Autodesk Fusion 360 part; units mm, degrees
note: some values were not read from the file. Chosen so that the rebuilt part matches the saved one: a direction. Set by a fixed rule: which sketch regions a step uses; which face or edge a step refers to.
(part 5 of 6)
  line L1273 (135.5672, -17.489) -> (135.5672, -15.9015)
  spline S993 degree 3 poles (135.5672, -15.9015) (135.5672, -15.8869) (135.5553, -15.875) (135.5408, -15.875) knots 0 0 0 0 1 1 1 1
  line L1274 (135.5408, -15.875) -> (135.1703, -15.875)
  spline S994 degree 3 poles (135.1703, -15.875) (135.1439, -15.875) (135.1703, -15.9015) (135.1703, -15.875) knots 0 0 0 0 1 1 1 1
  line L1275 (135.1703, -15.875) -> (135.1703, -14.3404)
  spline S995 degree 3 poles (135.1703, -14.3404) (135.1703, -14.314) (135.1439, -14.3404) (135.1703, -14.3404) knots 0 0 0 0 1 1 1 1
  line L1276 (135.1703, -14.3404) -> (135.5408, -14.3404)
  spline S996 degree 3 poles (135.5408, -14.3404) (135.5553, -14.3404) (135.5672, -14.3285) (135.5672, -14.314) knots 0 0 0 0 1 1 1 1
  line L1277 (135.5672, -14.314) -> (135.5672, -12.7265)
  spline S997 degree 3 poles (135.5672, -12.7265) (135.5672, -12.7119) (135.5553, -12.7) (135.5408, -12.7) knots 0 0 0 0 1 1 1 1
  line L1278 (135.5408, -12.7) -> (135.1703, -12.7)
  spline S998 degree 3 poles (135.1703, -12.7) (135.1439, -12.7) (135.1703, -12.7265) (135.1703, -12.7) knots 0 0 0 0 1 1 1 1
  line L1279 (135.1703, -12.7) -> (135.1703, -11.1654)
  spline S999 degree 3 poles (135.1703, -11.1654) (135.1703, -11.139) (135.1439, -11.1654) (135.1703, -11.1654) knots 0 0 0 0 1 1 1 1
  line L1280 (135.1703, -11.1654) -> (135.5408, -11.1654)
  spline S1000 degree 3 poles (135.5408, -11.1654) (135.5553, -11.1654) (135.5672, -11.1535) (135.5672, -11.139) knots 0 0 0 0 1 1 1 1
  line L1281 (135.5672, -11.139) -> (135.5672, -9.5515)
  spline S1001 degree 3 poles (135.5672, -9.5515) (135.5672, -9.5369) (135.5553, -9.525) (135.5408, -9.525) knots 0 0 0 0 1 1 1 1
  line L1282 (135.5408, -9.525) -> (135.1703, -9.525)
  spline S1002 degree 3 poles (135.1703, -9.525) (135.1439, -9.525) (135.1703, -9.5515) (135.1703, -9.525) knots 0 0 0 0 1 1 1 1
  line L1283 (135.1703, -9.525) -> (135.1703, -7.9904)
  spline S1003 degree 3 poles (135.1703, -7.9904) (135.1703, -7.964) (135.1439, -7.9904) (135.1703, -7.9904) knots 0 0 0 0 1 1 1 1
  line L1284 (135.1703, -7.9904) -> (135.5408, -7.9904)
  spline S1004 degree 3 poles (135.5408, -7.9904) (135.5553, -7.9904) (135.5672, -7.9785) (135.5672, -7.964) knots 0 0 0 0 1 1 1 1
  line L1285 (135.5672, -7.964) -> (135.5672, -6.3765)
  spline S1005 degree 3 poles (135.5672, -6.3765) (135.5672, -6.3619) (135.5553, -6.35) (135.5408, -6.35) knots 0 0 0 0 1 1 1 1
  line L1286 (135.5408, -6.35) -> (135.1703, -6.35)
  spline S1006 degree 3 poles (135.1703, -6.35) (135.1439, -6.35) (135.1703, -6.3765) (135.1703, -6.35) knots 0 0 0 0 1 1 1 1
  line L1287 (135.1703, -6.35) -> (135.1703, -3.466)
  spline S1007 degree 3 poles (135.1703, -3.466) (135.1703, -3.4515) (135.1584, -3.4396) (135.1439, -3.4396) knots 0 0 0 0 1 1 1 1
  line L1288 (135.1439, -3.4396) -> (135.328, -3.4396)
  line L1289 (135.328, -3.4396) -> (133.9226, -3.4396)
  spline S1008 degree 3 poles (133.9226, -3.4396) (133.8961, -3.4396) (133.9226, -3.466) (133.9226, -3.4396) knots 0 0 0 0 1 1 1 1
  line L1290 (133.9226, -3.4396) -> (133.9226, -2.6723)
  spline S1009 degree 3 poles (133.9226, -2.6723) (133.9226, -2.6577) (133.9109, -2.6458) (133.8961, -2.6458) knots 0 0 0 0 1 1 1 1
  line L1291 (133.8961, -2.6458) -> (132.3086, -2.6458)
  spline S1010 degree 3 poles (132.3086, -2.6458) (132.294, -2.6458) (132.2821, -2.6577) (132.2821, -2.6723) knots 0 0 0 0 1 1 1 1
  line L1292 (132.2821, -2.6723) -> (132.2821, -3.4396)
  spline S1011 degree 3 poles (132.2821, -3.4396) (132.2821, -3.466) (132.3086, -3.4396) (132.2821, -3.4396) knots 0 0 0 0 1 1 1 1
  line L1293 (132.2821, -3.4396) -> (130.8769, -3.4396)
  line L1294 (130.8769, -3.4396) -> (130.6642, -3.4396)
  spline S1012 degree 3 poles (130.6642, -3.4396) (130.6497, -3.4396) (130.6378, -3.4515) (130.6378, -3.466) knots 0 0 0 0 1 1 1 1
  line L1295 (130.6378, -3.466) -> (130.6378, -6.3765)
  spline S1013 degree 3 poles (130.6378, -6.3765) (130.6378, -6.391) (130.6497, -6.4029) (130.6642, -6.4029) knots 0 0 0 0 1 1 1 1
  line L1296 (130.6642, -6.4029) -> (131.0346, -6.4029)
  spline S1014 degree 3 poles (131.0346, -6.4029) (131.0611, -6.4029) (131.0346, -6.3765) (131.0346, -6.4029) knots 0 0 0 0 1 1 1 1
  line L1297 (131.0346, -6.4029) -> (131.0346, -7.9375)
  spline S1015 degree 3 poles (131.0346, -7.9375) (131.0346, -7.964) (131.0611, -7.9375) (131.0346, -7.9375) knots 0 0 0 0 1 1 1 1
  line L1298 (131.0346, -7.9375) -> (130.6642, -7.9375)
  spline S1016 degree 3 poles (130.6642, -7.9375) (130.6497, -7.9375) (130.6378, -7.9494) (130.6378, -7.964) knots 0 0 0 0 1 1 1 1
  line L1299 (130.6378, -7.964) -> (130.6378, -9.5515)
  spline S1017 degree 3 poles (130.6378, -9.5515) (130.6378, -9.566) (130.6497, -9.5779) (130.6642, -9.5779) knots 0 0 0 0 1 1 1 1
  line L1300 (130.6642, -9.5779) -> (131.0346, -9.5779)
  spline S1018 degree 3 poles (131.0346, -9.5779) (131.0611, -9.5779) (131.0346, -9.5515) (131.0346, -9.5779) knots 0 0 0 0 1 1 1 1
  line L1301 (131.0346, -9.5779) -> (131.0346, -11.1125)
  spline S1019 degree 3 poles (131.0346, -11.1125) (131.0346, -11.139) (131.0611, -11.1125) (131.0346, -11.1125) knots 0 0 0 0 1 1 1 1
  line L1302 (131.0346, -11.1125) -> (130.6642, -11.1125)
  spline S1020 degree 3 poles (130.6642, -11.1125) (130.6497, -11.1125) (130.6378, -11.1244) (130.6378, -11.139) knots 0 0 0 0 1 1 1 1
  line L1303 (130.6378, -11.139) -> (130.6378, -12.7265)
  spline S1021 degree 3 poles (130.6378, -12.7265) (130.6378, -12.741) (130.6497, -12.7529) (130.6642, -12.7529) knots 0 0 0 0 1 1 1 1
  line L1304 (130.6642, -12.7529) -> (131.0346, -12.7529)
  spline S1022 degree 3 poles (131.0346, -12.7529) (131.0611, -12.7529) (131.0346, -12.7265) (131.0346, -12.7529) knots 0 0 0 0 1 1 1 1
  line L1305 (131.0346, -12.7529) -> (131.0346, -14.2875)
  spline S1023 degree 3 poles (131.0346, -14.2875) (131.0346, -14.314) (131.0611, -14.2875) (131.0346, -14.2875) knots 0 0 0 0 1 1 1 1
  line L1306 (131.0346, -14.2875) -> (130.6642, -14.2875)
  spline S1024 degree 3 poles (130.6642, -14.2875) (130.6497, -14.2875) (130.6378, -14.2994) (130.6378, -14.314) knots 0 0 0 0 1 1 1 1
  line L1307 (130.6378, -14.314) -> (130.6378, -15.9015)
  spline S1025 degree 3 poles (130.6378, -15.9015) (130.6378, -15.916) (130.6497, -15.9279) (130.6642, -15.9279) knots 0 0 0 0 1 1 1 1
  line L1308 (130.6642, -15.9279) -> (131.0346, -15.9279)
  spline S1026 degree 3 poles (131.0346, -15.9279) (131.0611, -15.9279) (131.0346, -15.9015) (131.0346, -15.9279) knots 0 0 0 0 1 1 1 1
  line L1309 (131.0346, -15.9279) -> (131.0346, -17.4625)
  spline S1027 degree 3 poles (131.0346, -17.4625) (131.0346, -17.489) (131.0611, -17.4625) (131.0346, -17.4625) knots 0 0 0 0 1 1 1 1
  line L1310 (131.0346, -17.4625) -> (130.6642, -17.4625)
  spline S1028 degree 3 poles (130.6642, -17.4625) (130.6497, -17.4625) (130.6378, -17.4744) (130.6378, -17.489) knots 0 0 0 0 1 1 1 1
  line L1311 (130.6378, -17.489) -> (130.6378, -19.0765)
  spline S1029 degree 3 poles (130.6378, -19.0765) (130.6378, -19.091) (130.6497, -19.1029) (130.6642, -19.1029) knots 0 0 0 0 1 1 1 1
  line L1312 (130.6642, -19.1029) -> (131.0346, -19.1029)
  spline S1030 degree 3 poles (131.0346, -19.1029) (131.0611, -19.1029) (131.0346, -19.0765) (131.0346, -19.1029) knots 0 0 0 0 1 1 1 1
  line L1313 (131.0346, -19.1029) -> (131.0346, -20.6375)
  spline S1031 degree 3 poles (131.0346, -20.6375) (131.0346, -20.664) (131.0611, -20.6375) (131.0346, -20.6375) knots 0 0 0 0 1 1 1 1
  line L1314 (131.0346, -20.6375) -> (130.6642, -20.6375)
  spline S1032 degree 3 poles (130.6642, -20.6375) (130.6497, -20.6375) (130.6378, -20.6494) (130.6378, -20.664) knots 0 0 0 0 1 1 1 1
  line L1315 (130.6378, -20.664) -> (130.6378, -22.2515)
  spline S1033 degree 3 poles (130.6378, -22.2515) (130.6378, -22.266) (130.6497, -22.2779) (130.6642, -22.2779) knots 0 0 0 0 1 1 1 1
  line L1316 (130.6642, -22.2779) -> (131.0346, -22.2779)
  spline S1034 degree 3 poles (131.0346, -22.2779) (131.0611, -22.2779) (131.0346, -22.2515) (131.0346, -22.2779) knots 0 0 0 0 1 1 1 1
  line L1317 (131.0346, -22.2779) -> (131.0346, -23.8125)
  spline S1035 degree 3 poles (131.0346, -23.8125) (131.0346, -23.839) (131.0611, -23.8125) (131.0346, -23.8125) knots 0 0 0 0 1 1 1 1
  line L1318 (131.0346, -23.8125) -> (130.6642, -23.8125)
  spline S1036 degree 3 poles (130.6642, -23.8125) (130.6497, -23.8125) (130.6378, -23.8244) (130.6378, -23.839) knots 0 0 0 0 1 1 1 1
  line L1319 (130.6378, -23.839) -> (130.6378, -25.4265)
  spline S1037 degree 3 poles (130.6378, -25.4265) (130.6378, -25.441) (130.6497, -25.4529) (130.6642, -25.4529) knots 0 0 0 0 1 1 1 1
  line L1320 (130.6642, -25.4529) -> (131.0346, -25.4529)
  spline S1038 degree 3 poles (131.0346, -25.4529) (131.0611, -25.4529) (131.0346, -25.4265) (131.0346, -25.4529) knots 0 0 0 0 1 1 1 1
  line L1321 (131.0346, -25.4529) -> (131.0346, -26.9875)
  spline S1039 degree 3 poles (131.0346, -26.9875) (131.0346, -27.014) (131.0611, -26.9875) (131.0346, -26.9875) knots 0 0 0 0 1 1 1 1
  line L1322 (131.0346, -26.9875) -> (130.6642, -26.9875)
  spline S1040 degree 3 poles (130.6642, -26.9875) (130.6497, -26.9875) (130.6378, -26.9994) (130.6378, -27.014) knots 0 0 0 0 1 1 1 1
  line L1323 (130.6378, -27.014) -> (130.6378, -29.9244)
  spline S1041 degree 3 poles (130.6378, -29.9244) (130.6378, -29.9389) (130.6497, -29.9508) (130.6642, -29.9508) knots 0 0 0 0 1 1 1 1
  line L1324 (130.6642, -29.9508) -> (130.8769, -29.9508)
  line L1325 (136.2033, -29.9508) -> (137.6085, -29.9508)
  spline S1042 degree 3 poles (137.6085, -29.9508) (137.6349, -29.9508) (137.6085, -29.9244) (137.6085, -29.9508) knots 0 0 0 0 1 1 1 1
  line L1326 (137.6085, -29.9508) -> (137.6085, -30.7181)
  spline S1043 degree 3 poles (137.6085, -30.7181) (137.6085, -30.7327) (137.6204, -30.7446) (137.6349, -30.7446) knots 0 0 0 0 1 1 1 1
  line L1327 (137.6349, -30.7446) -> (139.2224, -30.7446)
  spline S1044 degree 3 poles (139.2224, -30.7446) (139.237, -30.7446) (139.2489, -30.7327) (139.2489, -30.7181) knots 0 0 0 0 1 1 1 1
  line L1328 (139.2489, -30.7181) -> (139.2489, -29.9508)
  spline S1045 degree 3 poles (139.2489, -29.9508) (139.2489, -29.9244) (139.2224, -29.9508) (139.2489, -29.9508) knots 0 0 0 0 1 1 1 1
  line L1329 (139.2489, -29.9508) -> (140.6544, -29.9508)
  line L1330 (140.6544, -29.9508) -> (140.5533, -29.9508)
  spline S1046 degree 3 poles (140.5533, -29.9508) (140.5681, -29.9508) (140.5797, -29.9389) (140.5797, -29.9244) knots 0 0 0 0 1 1 1 1
  line L1331 (140.5797, -29.9244) -> (140.5797, -27.0404)
  spline S1047 degree 3 poles (140.5797, -27.0404) (140.5797, -27.014) (140.5533, -27.0404) (140.5797, -27.0404) knots 0 0 0 0 1 1 1 1
  line L1332 (140.5797, -27.0404) -> (140.7589, -27.0404)
  spline S1048 degree 3 poles (140.7589, -27.0404) (140.7734, -27.0404) (140.7853, -27.0285) (140.7853, -27.014) knots 0 0 0 0 1 1 1 1
  line L1333 (140.7853, -27.014) -> (140.7853, -25.4265)
  spline S1049 degree 3 poles (140.7853, -25.4265) (140.7853, -25.4119) (140.7734, -25.4) (140.7589, -25.4) knots 0 0 0 0 1 1 1 1
  line L1334 (140.7589, -25.4) -> (140.5797, -25.4)
  spline S1050 degree 3 poles (140.5797, -25.4) (140.5533, -25.4) (140.5797, -25.4265) (140.5797, -25.4) knots 0 0 0 0 1 1 1 1
  line L1335 (140.5797, -25.4) -> (140.5797, -23.8654)
  spline S1051 degree 3 poles (140.5797, -23.8654) (140.5797, -23.839) (140.5533, -23.8654) (140.5797, -23.8654) knots 0 0 0 0 1 1 1 1
  line L1336 (140.5797, -23.8654) -> (140.7589, -23.8654)
  spline S1052 degree 3 poles (140.7589, -23.8654) (140.7734, -23.8654) (140.7853, -23.8535) (140.7853, -23.839) knots 0 0 0 0 1 1 1 1
  line L1337 (140.7853, -23.839) -> (140.7853, -22.2515)
  spline S1053 degree 3 poles (140.7853, -22.2515) (140.7853, -22.2369) (140.7734, -22.225) (140.7589, -22.225) knots 0 0 0 0 1 1 1 1
  line L1338 (140.7589, -22.225) -> (140.5797, -22.225)
  spline S1054 degree 3 poles (140.5797, -22.225) (140.5533, -22.225) (140.5797, -22.2515) (140.5797, -22.225) knots 0 0 0 0 1 1 1 1
  line L1339 (140.5797, -22.225) -> (140.5797, -20.6904)
  spline S1055 degree 3 poles (140.5797, -20.6904) (140.5797, -20.664) (140.5533, -20.6904) (140.5797, -20.6904) knots 0 0 0 0 1 1 1 1
  line L1340 (140.5797, -20.6904) -> (140.7589, -20.6904)
  spline S1056 degree 3 poles (140.7589, -20.6904) (140.7734, -20.6904) (140.7853, -20.6785) (140.7853, -20.664) knots 0 0 0 0 1 1 1 1
  line L1341 (140.7853, -20.664) -> (140.7853, -19.0765)
  spline S1057 degree 3 poles (140.7853, -19.0765) (140.7853, -19.0619) (140.7734, -19.05) (140.7589, -19.05) knots 0 0 0 0 1 1 1 1
  line L1342 (140.7589, -19.05) -> (140.5797, -19.05)
  spline S1058 degree 3 poles (140.5797, -19.05) (140.5533, -19.05) (140.5797, -19.0765) (140.5797, -19.05) knots 0 0 0 0 1 1 1 1
  line L1343 (140.5797, -19.05) -> (140.5797, -17.5154)
  spline S1059 degree 3 poles (140.5797, -17.5154) (140.5797, -17.489) (140.5533, -17.5154) (140.5797, -17.5154) knots 0 0 0 0 1 1 1 1
  line L1344 (140.5797, -17.5154) -> (140.7589, -17.5154)
  spline S1060 degree 3 poles (140.7589, -17.5154) (140.7734, -17.5154) (140.7853, -17.5035) (140.7853, -17.489) knots 0 0 0 0 1 1 1 1
  line L1345 (140.7853, -17.489) -> (140.7853, -15.9015)
  spline S1061 degree 3 poles (140.7853, -15.9015) (140.7853, -15.8869) (140.7734, -15.875) (140.7589, -15.875) knots 0 0 0 0 1 1 1 1
  line L1346 (140.7589, -15.875) -> (140.5797, -15.875)
  spline S1062 degree 3 poles (140.5797, -15.875) (140.5533, -15.875) (140.5797, -15.9015) (140.5797, -15.875) knots 0 0 0 0 1 1 1 1
  line L1347 (140.5797, -15.875) -> (140.5797, -14.3404)
  spline S1063 degree 3 poles (140.5797, -14.3404) (140.5797, -14.314) (140.5533, -14.3404) (140.5797, -14.3404) knots 0 0 0 0 1 1 1 1
  line L1348 (140.5797, -14.3404) -> (140.7589, -14.3404)
  spline S1064 degree 3 poles (140.7589, -14.3404) (140.7734, -14.3404) (140.7853, -14.3285) (140.7853, -14.314) knots 0 0 0 0 1 1 1 1
  line L1349 (140.7853, -14.314) -> (140.7853, -12.7265)
  spline S1065 degree 3 poles (140.7853, -12.7265) (140.7853, -12.7119) (140.7734, -12.7) (140.7589, -12.7) knots 0 0 0 0 1 1 1 1
  line L1350 (140.7589, -12.7) -> (140.5797, -12.7)
  spline S1066 degree 3 poles (140.5797, -12.7) (140.5533, -12.7) (140.5797, -12.7265) (140.5797, -12.7) knots 0 0 0 0 1 1 1 1
  line L1351 (140.5797, -12.7) -> (140.5797, -11.1654)
  spline S1067 degree 3 poles (140.5797, -11.1654) (140.5797, -11.139) (140.5533, -11.1654) (140.5797, -11.1654) knots 0 0 0 0 1 1 1 1
  line L1352 (140.5797, -11.1654) -> (140.7589, -11.1654)
  spline S1068 degree 3 poles (140.7589, -11.1654) (140.7734, -11.1654) (140.7853, -11.1535) (140.7853, -11.139) knots 0 0 0 0 1 1 1 1
  line L1353 (140.7853, -11.139) -> (140.7853, -9.5515)
  spline S1069 degree 3 poles (140.7853, -9.5515) (140.7853, -9.5369) (140.7734, -9.525) (140.7589, -9.525) knots 0 0 0 0 1 1 1 1
  line L1354 (140.7589, -9.525) -> (140.5797, -9.525)
  spline S1070 degree 3 poles (140.5797, -9.525) (140.5533, -9.525) (140.5797, -9.5515) (140.5797, -9.525) knots 0 0 0 0 1 1 1 1
  line L1355 (140.5797, -9.525) -> (140.5797, -7.9904)
  spline S1071 degree 3 poles (140.5797, -7.9904) (140.5797, -7.964) (140.5533, -7.9904) (140.5797, -7.9904) knots 0 0 0 0 1 1 1 1
  line L1356 (140.5797, -7.9904) -> (140.7589, -7.9904)
  spline S1072 degree 3 poles (140.7589, -7.9904) (140.7734, -7.9904) (140.7853, -7.9785) (140.7853, -7.964) knots 0 0 0 0 1 1 1 1
  line L1357 (140.7853, -7.964) -> (140.7853, -6.3765)
  spline S1073 degree 3 poles (140.7853, -6.3765) (140.7853, -6.3619) (140.7734, -6.35) (140.7589, -6.35) knots 0 0 0 0 1 1 1 1
  line L1358 (140.7589, -6.35) -> (140.5797, -6.35)
  spline S1074 degree 3 poles (140.5797, -6.35) (140.5533, -6.35) (140.5797, -6.3765) (140.5797, -6.35) knots 0 0 0 0 1 1 1 1
  line L1359 (140.5797, -6.35) -> (140.5797, -3.466)
  spline S1075 degree 3 poles (140.5797, -3.466) (140.5797, -3.4515) (140.5681, -3.4396) (140.5533, -3.4396) knots 0 0 0 0 1 1 1 1
  line L1360 (140.5533, -3.4396) -> (140.6544, -3.4396)
  line L1361 (140.6544, -3.4396) -> (139.2489, -3.4396)
  spline S1076 degree 3 poles (139.2489, -3.4396) (139.2224, -3.4396) (139.2489, -3.466) (139.2489, -3.4396) knots 0 0 0 0 1 1 1 1
  line L1362 (139.2489, -3.4396) -> (139.2489, -2.6723)
  spline S1077 degree 3 poles (139.2489, -2.6723) (139.2489, -2.6577) (139.237, -2.6458) (139.2224, -2.6458) knots 0 0 0 0 1 1 1 1
  line L1363 (139.2224, -2.6458) -> (137.6349, -2.6458)
  spline S1078 degree 3 poles (137.6349, -2.6458) (137.6204, -2.6458) (137.6085, -2.6577) (137.6085, -2.6723) knots 0 0 0 0 1 1 1 1
  line L1364 (137.6085, -2.6723) -> (137.6085, -3.4396)
  spline S1079 degree 3 poles (137.6085, -3.4396) (137.6085, -3.466) (137.6349, -3.4396) (137.6085, -3.4396) knots 0 0 0 0 1 1 1 1
  line L1365 (137.6085, -3.4396) -> (136.2033, -3.4396)
  line L1366 (136.2033, -3.4396) -> (135.9905, -3.4396)
  spline S1080 degree 3 poles (135.9905, -3.4396) (135.976, -3.4396) (135.9641, -3.4515) (135.9641, -3.466) knots 0 0 0 0 1 1 1 1
  line L1367 (135.9641, -3.466) -> (135.9641, -6.3765)
  spline S1081 degree 3 poles (135.9641, -6.3765) (135.9641, -6.391) (135.976, -6.4029) (135.9905, -6.4029) knots 0 0 0 0 1 1 1 1
  line L1368 (135.9905, -6.4029) -> (136.361, -6.4029)
  spline S1082 degree 3 poles (136.361, -6.4029) (136.3874, -6.4029) (136.361, -6.3765) (136.361, -6.4029) knots 0 0 0 0 1 1 1 1
  line L1369 (136.361, -6.4029) -> (136.361, -7.9375)
  spline S1083 degree 3 poles (136.361, -7.9375) (136.361, -7.964) (136.3874, -7.9375) (136.361, -7.9375) knots 0 0 0 0 1 1 1 1
  line L1370 (136.361, -7.9375) -> (135.9905, -7.9375)
  spline S1084 degree 3 poles (135.9905, -7.9375) (135.976, -7.9375) (135.9641, -7.9494) (135.9641, -7.964) knots 0 0 0 0 1 1 1 1
  line L1371 (135.9641, -7.964) -> (135.9641, -9.5515)
  spline S1085 degree 3 poles (135.9641, -9.5515) (135.9641, -9.566) (135.976, -9.5779) (135.9905, -9.5779) knots 0 0 0 0 1 1 1 1
  line L1372 (135.9905, -9.5779) -> (136.361, -9.5779)
  spline S1086 degree 3 poles (136.361, -9.5779) (136.3874, -9.5779) (136.361, -9.5515) (136.361, -9.5779) knots 0 0 0 0 1 1 1 1
  line L1373 (136.361, -9.5779) -> (136.361, -11.1125)
  spline S1087 degree 3 poles (136.361, -11.1125) (136.361, -11.139) (136.3874, -11.1125) (136.361, -11.1125) knots 0 0 0 0 1 1 1 1
  line L1374 (136.361, -11.1125) -> (135.9905, -11.1125)
  spline S1088 degree 3 poles (135.9905, -11.1125) (135.976, -11.1125) (135.9641, -11.1244) (135.9641, -11.139) knots 0 0 0 0 1 1 1 1
  line L1375 (135.9641, -11.139) -> (135.9641, -12.7265)
  spline S1089 degree 3 poles (135.9641, -12.7265) (135.9641, -12.741) (135.976, -12.7529) (135.9905, -12.7529) knots 0 0 0 0 1 1 1 1
  line L1376 (135.9905, -12.7529) -> (136.361, -12.7529)
  spline S1090 degree 3 poles (136.361, -12.7529) (136.3874, -12.7529) (136.361, -12.7265) (136.361, -12.7529) knots 0 0 0 0 1 1 1 1
  line L1377 (136.361, -12.7529) -> (136.361, -14.2875)
  spline S1091 degree 3 poles (136.361, -14.2875) (136.361, -14.314) (136.3874, -14.2875) (136.361, -14.2875) knots 0 0 0 0 1 1 1 1
  line L1378 (136.361, -14.2875) -> (135.9905, -14.2875)
  spline S1092 degree 3 poles (135.9905, -14.2875) (135.976, -14.2875) (135.9641, -14.2994) (135.9641, -14.314) knots 0 0 0 0 1 1 1 1
  line L1379 (135.9641, -14.314) -> (135.9641, -15.9015)
  spline S1093 degree 3 poles (135.9641, -15.9015) (135.9641, -15.916) (135.976, -15.9279) (135.9905, -15.9279) knots 0 0 0 0 1 1 1 1
  line L1380 (135.9905, -15.9279) -> (136.361, -15.9279)
  spline S1094 degree 3 poles (136.361, -15.9279) (136.3874, -15.9279) (136.361, -15.9015) (136.361, -15.9279) knots 0 0 0 0 1 1 1 1
  line L1381 (136.361, -15.9279) -> (136.361, -17.4625)
  spline S1095 degree 3 poles (136.361, -17.4625) (136.361, -17.489) (136.3874, -17.4625) (136.361, -17.4625) knots 0 0 0 0 1 1 1 1
  line L1382 (136.361, -17.4625) -> (135.9905, -17.4625)
  spline S1096 degree 3 poles (135.9905, -17.4625) (135.976, -17.4625) (135.9641, -17.4744) (135.9641, -17.489) knots 0 0 0 0 1 1 1 1
  line L1383 (135.9641, -17.489) -> (135.9641, -19.0765)
  spline S1097 degree 3 poles (135.9641, -19.0765) (135.9641, -19.091) (135.976, -19.1029) (135.9905, -19.1029) knots 0 0 0 0 1 1 1 1
  line L1384 (135.9905, -19.1029) -> (136.361, -19.1029)
  spline S1098 degree 3 poles (136.361, -19.1029) (136.3874, -19.1029) (136.361, -19.0765) (136.361, -19.1029) knots 0 0 0 0 1 1 1 1
  line L1385 (136.361, -19.1029) -> (136.361, -20.6375)
  spline S1099 degree 3 poles (136.361, -20.6375) (136.361, -20.664) (136.3874, -20.6375) (136.361, -20.6375) knots 0 0 0 0 1 1 1 1
  line L1386 (136.361, -20.6375) -> (135.9905, -20.6375)
  spline S1100 degree 3 poles (135.9905, -20.6375) (135.976, -20.6375) (135.9641, -20.6494) (135.9641, -20.664) knots 0 0 0 0 1 1 1 1
  line L1387 (135.9641, -20.664) -> (135.9641, -22.2515)
  spline S1101 degree 3 poles (135.9641, -22.2515) (135.9641, -22.266) (135.976, -22.2779) (135.9905, -22.2779) knots 0 0 0 0 1 1 1 1
  line L1388 (135.9905, -22.2779) -> (136.361, -22.2779)
  spline S1102 degree 3 poles (136.361, -22.2779) (136.3874, -22.2779) (136.361, -22.2515) (136.361, -22.2779) knots 0 0 0 0 1 1 1 1
  line L1389 (136.361, -22.2779) -> (136.361, -23.8125)
  spline S1103 degree 3 poles (136.361, -23.8125) (136.361, -23.839) (136.3874, -23.8125) (136.361, -23.8125) knots 0 0 0 0 1 1 1 1
  line L1390 (136.361, -23.8125) -> (135.9905, -23.8125)
  spline S1104 degree 3 poles (135.9905, -23.8125) (135.976, -23.8125) (135.9641, -23.8244) (135.9641, -23.839) knots 0 0 0 0 1 1 1 1
  line L1391 (135.9641, -23.839) -> (135.9641, -25.4265)
  spline S1105 degree 3 poles (135.9641, -25.4265) (135.9641, -25.441) (135.976, -25.4529) (135.9905, -25.4529) knots 0 0 0 0 1 1 1 1
  line L1392 (135.9905, -25.4529) -> (136.361, -25.4529)
  spline S1106 degree 3 poles (136.361, -25.4529) (136.3874, -25.4529) (136.361, -25.4265) (136.361, -25.4529) knots 0 0 0 0 1 1 1 1
  line L1393 (136.361, -25.4529) -> (136.361, -26.9875)
  spline S1107 degree 3 poles (136.361, -26.9875) (136.361, -27.014) (136.3874, -26.9875) (136.361, -26.9875) knots 0 0 0 0 1 1 1 1
  line L1394 (136.361, -26.9875) -> (135.9905, -26.9875)
  spline S1108 degree 3 poles (135.9905, -26.9875) (135.976, -26.9875) (135.9641, -26.9994) (135.9641, -27.014) knots 0 0 0 0 1 1 1 1
  line L1395 (135.9641, -27.014) -> (135.9641, -29.9244)
  spline S1109 degree 3 poles (135.9641, -29.9244) (135.9641, -29.9389) (135.976, -29.9508) (135.9905, -29.9508) knots 0 0 0 0 1 1 1 1
  line L1396 (135.9905, -29.9508) -> (136.2033, -29.9508)
  line L1397 (141.3132, -29.9508) -> (143.1388, -29.9508)
  spline S1110 degree 3 poles (143.1388, -29.9508) (143.1652, -29.9508) (143.1388, -29.9244) (143.1388, -29.9508) knots 0 0 0 0 1 1 1 1
  line L1398 (143.1388, -29.9508) -> (143.1388, -30.7181)
  spline S1111 degree 3 poles (143.1388, -30.7181) (143.1388, -30.7327) (143.1507, -30.7446) (143.1652, -30.7446) knots 0 0 0 0 1 1 1 1
  line L1399 (143.1652, -30.7446) -> (144.7527, -30.7446)
  spline S1112 degree 3 poles (144.7527, -30.7446) (144.7673, -30.7446) (144.7792, -30.7327) (144.7792, -30.7181) knots 0 0 0 0 1 1 1 1
  line L1400 (144.7792, -30.7181) -> (144.7792, -29.9508)
  spline S1113 degree 3 poles (144.7792, -29.9508) (144.7792, -29.9244) (144.7527, -29.9508) (144.7792, -29.9508) knots 0 0 0 0 1 1 1 1
  line L1401 (144.7792, -29.9508) -> (146.6048, -29.9508)
  spline S1114 degree 3 poles (146.6048, -29.9508) (146.6194, -29.9508) (146.6313, -29.9389) (146.6313, -29.9244) knots 0 0 0 0 1 1 1 1
  line L1402 (146.6313, -29.9244) -> (146.6313, -3.466)
  spline S1115 degree 3 poles (146.6313, -3.466) (146.6313, -3.4515) (146.6194, -3.4396) (146.6048, -3.4396) knots 0 0 0 0 1 1 1 1
  line L1403 (146.6048, -3.4396) -> (144.7792, -3.4396)
  spline S1116 degree 3 poles (144.7792, -3.4396) (144.7527, -3.4396) (144.7792, -3.466) (144.7792, -3.4396) knots 0 0 0 0 1 1 1 1
  line L1404 (144.7792, -3.4396) -> (144.7792, -2.6723)
  spline S1117 degree 3 poles (144.7792, -2.6723) (144.7792, -2.6577) (144.7673, -2.6458) (144.7527, -2.6458) knots 0 0 0 0 1 1 1 1
  line L1405 (144.7527, -2.6458) -> (143.1652, -2.6458)
  spline S1118 degree 3 poles (143.1652, -2.6458) (143.1507, -2.6458) (143.1388, -2.6577) (143.1388, -2.6723) knots 0 0 0 0 1 1 1 1
  line L1406 (143.1388, -2.6723) -> (143.1388, -3.4396)
  spline S1119 degree 3 poles (143.1388, -3.4396) (143.1388, -3.466) (143.1652, -3.4396) (143.1388, -3.4396) knots 0 0 0 0 1 1 1 1
  line L1407 (143.1388, -3.4396) -> (141.3132, -3.4396)
  line L1408 (141.3132, -3.4396) -> (141.2087, -3.4396)
  spline S1120 degree 3 poles (141.2087, -3.4396) (141.1941, -3.4396) (141.1822, -3.4515) (141.1822, -3.466) knots 0 0 0 0 1 1 1 1
  line L1409 (141.1822, -3.466) -> (141.1822, -6.3765)
  spline S1121 degree 3 poles (141.1822, -6.3765) (141.1822, -6.391) (141.1941, -6.4029) (141.2087, -6.4029) knots 0 0 0 0 1 1 1 1
  line L1410 (141.2087, -6.4029) -> (141.3875, -6.4029)
  spline S1122 degree 3 poles (141.3875, -6.4029) (141.414, -6.4029) (141.3875, -6.3765) (141.3875, -6.4029) knots 0 0 0 0 1 1 1 1
  line L1411 (141.3875, -6.4029) -> (141.3875, -7.9375)
  spline S1123 degree 3 poles (141.3875, -7.9375) (141.3875, -7.964) (141.414, -7.9375) (141.3875, -7.9375) knots 0 0 0 0 1 1 1 1
  line L1412 (141.3875, -7.9375) -> (141.2087, -7.9375)
  spline S1124 degree 3 poles (141.2087, -7.9375) (141.1941, -7.9375) (141.1822, -7.9494) (141.1822, -7.964) knots 0 0 0 0 1 1 1 1
  line L1413 (141.1822, -7.964) -> (141.1822, -9.5515)
  spline S1125 degree 3 poles (141.1822, -9.5515) (141.1822, -9.566) (141.1941, -9.5779) (141.2087, -9.5779) knots 0 0 0 0 1 1 1 1
  line L1414 (141.2087, -9.5779) -> (141.3875, -9.5779)
  spline S1126 degree 3 poles (141.3875, -9.5779) (141.414, -9.5779) (141.3875, -9.5515) (141.3875, -9.5779) knots 0 0 0 0 1 1 1 1
  line L1415 (141.3875, -9.5779) -> (141.3875, -11.1125)
  spline S1127 degree 3 poles (141.3875, -11.1125) (141.3875, -11.139) (141.414, -11.1125) (141.3875, -11.1125) knots 0 0 0 0 1 1 1 1
  line L1416 (141.3875, -11.1125) -> (141.2087, -11.1125)
  spline S1128 degree 3 poles (141.2087, -11.1125) (141.1941, -11.1125) (141.1822, -11.1244) (141.1822, -11.139) knots 0 0 0 0 1 1 1 1
  line L1417 (141.1822, -11.139) -> (141.1822, -12.7265)
  spline S1129 degree 3 poles (141.1822, -12.7265) (141.1822, -12.741) (141.1941, -12.7529) (141.2087, -12.7529) knots 0 0 0 0 1 1 1 1
  line L1418 (141.2087, -12.7529) -> (141.3875, -12.7529)
  spline S1130 degree 3 poles (141.3875, -12.7529) (141.414, -12.7529) (141.3875, -12.7265) (141.3875, -12.7529) knots 0 0 0 0 1 1 1 1
  line L1419 (141.3875, -12.7529) -> (141.3875, -14.2875)
  spline S1131 degree 3 poles (141.3875, -14.2875) (141.3875, -14.314) (141.414, -14.2875) (141.3875, -14.2875) knots 0 0 0 0 1 1 1 1
  line L1420 (141.3875, -14.2875) -> (141.2087, -14.2875)
  spline S1132 degree 3 poles (141.2087, -14.2875) (141.1941, -14.2875) (141.1822, -14.2994) (141.1822, -14.314) knots 0 0 0 0 1 1 1 1
  line L1421 (141.1822, -14.314) -> (141.1822, -15.9015)
  spline S1133 degree 3 poles (141.1822, -15.9015) (141.1822, -15.916) (141.1941, -15.9279) (141.2087, -15.9279) knots 0 0 0 0 1 1 1 1
  line L1422 (141.2087, -15.9279) -> (141.3875, -15.9279)
  spline S1134 degree 3 poles (141.3875, -15.9279) (141.414, -15.9279) (141.3875, -15.9015) (141.3875, -15.9279) knots 0 0 0 0 1 1 1 1
  line L1423 (141.3875, -15.9279) -> (141.3875, -17.4625)
  spline S1135 degree 3 poles (141.3875, -17.4625) (141.3875, -17.489) (141.414, -17.4625) (141.3875, -17.4625) knots 0 0 0 0 1 1 1 1
  line L1424 (141.3875, -17.4625) -> (141.2087, -17.4625)
  spline S1136 degree 3 poles (141.2087, -17.4625) (141.1941, -17.4625) (141.1822, -17.4744) (141.1822, -17.489) knots 0 0 0 0 1 1 1 1
  line L1425 (141.1822, -17.489) -> (141.1822, -19.0765)
  spline S1137 degree 3 poles (141.1822, -19.0765) (141.1822, -19.091) (141.1941, -19.1029) (141.2087, -19.1029) knots 0 0 0 0 1 1 1 1
  line L1426 (141.2087, -19.1029) -> (141.3875, -19.1029)
  spline S1138 degree 3 poles (141.3875, -19.1029) (141.414, -19.1029) (141.3875, -19.0765) (141.3875, -19.1029) knots 0 0 0 0 1 1 1 1
  line L1427 (141.3875, -19.1029) -> (141.3875, -20.6375)
  spline S1139 degree 3 poles (141.3875, -20.6375) (141.3875, -20.664) (141.414, -20.6375) (141.3875, -20.6375) knots 0 0 0 0 1 1 1 1
  line L1428 (141.3875, -20.6375) -> (141.2087, -20.6375)
  spline S1140 degree 3 poles (141.2087, -20.6375) (141.1941, -20.6375) (141.1822, -20.6494) (141.1822, -20.664) knots 0 0 0 0 1 1 1 1
  line L1429 (141.1822, -20.664) -> (141.1822, -22.2515)
  spline S1141 degree 3 poles (141.1822, -22.2515) (141.1822, -22.266) (141.1941, -22.2779) (141.2087, -22.2779) knots 0 0 0 0 1 1 1 1
  line L1430 (141.2087, -22.2779) -> (141.3875, -22.2779)
  spline S1142 degree 3 poles (141.3875, -22.2779) (141.414, -22.2779) (141.3875, -22.2515) (141.3875, -22.2779) knots 0 0 0 0 1 1 1 1
  line L1431 (141.3875, -22.2779) -> (141.3875, -23.8125)
  spline S1143 degree 3 poles (141.3875, -23.8125) (141.3875, -23.839) (141.414, -23.8125) (141.3875, -23.8125) knots 0 0 0 0 1 1 1 1
  line L1432 (141.3875, -23.8125) -> (141.2087, -23.8125)
  spline S1144 degree 3 poles (141.2087, -23.8125) (141.1941, -23.8125) (141.1822, -23.8244) (141.1822, -23.839) knots 0 0 0 0 1 1 1 1
  line L1433 (141.1822, -23.839) -> (141.1822, -25.4265)
  spline S1145 degree 3 poles (141.1822, -25.4265) (141.1822, -25.441) (141.1941, -25.4529) (141.2087, -25.4529) knots 0 0 0 0 1 1 1 1
  line L1434 (141.2087, -25.4529) -> (141.3875, -25.4529)
  spline S1146 degree 3 poles (141.3875, -25.4529) (141.414, -25.4529) (141.3875, -25.4265) (141.3875, -25.4529) knots 0 0 0 0 1 1 1 1
  line L1435 (141.3875, -25.4529) -> (141.3875, -26.9875)
  spline S1147 degree 3 poles (141.3875, -26.9875) (141.3875, -27.014) (141.414, -26.9875) (141.3875, -26.9875) knots 0 0 0 0 1 1 1 1
  line L1436 (141.3875, -26.9875) -> (141.2087, -26.9875)
  spline S1148 degree 3 poles (141.2087, -26.9875) (141.1941, -26.9875) (141.1822, -26.9994) (141.1822, -27.014) knots 0 0 0 0 1 1 1 1
  line L1437 (141.1822, -27.014) -> (141.1822, -29.9244)
  spline S1149 degree 3 poles (141.1822, -29.9244) (141.1822, -29.9389) (141.1941, -29.9508) (141.2087, -29.9508) knots 0 0 0 0 1 1 1 1
  line L1438 (141.2087, -29.9508) -> (141.3132, -29.9508)
  line L1439 (15.9015, -59.69) -> (24.2653, -59.69) construction
  line L1440 (24.2653, -59.69) -> (24.2653, -57.0442) construction
  line L1441 (24.2653, -57.0442) -> (15.9015, -57.0442) construction
  line L1442 (15.9015, -57.0442) -> (15.9015, -59.69) construction
  line L1443 (43.9737, -2.6723) -> (2.6458, -2.6723)
  line L1444 (2.6458, -2.6723) -> (2.6458, -30.7181)
  line L1445 (2.6458, -30.7181) -> (43.9737, -30.7181)
  line L1446 (43.9737, -30.7181) -> (43.9737, -2.6723)
  line L1447 (2.6458, -2.6723) -> (2.6458, -30.7181)
  line L1448 (43.9737, -2.6723) -> (2.6458, -2.6723)
  line L1449 (43.9737, -30.7181) -> (43.9737, -2.6723)
  line L1450 (2.6458, -30.7181) -> (43.9737, -30.7181)
  point P0 (0.5, -4.6296)
  constraint horizontal L1443
  constraint vertical L1444
  constraint horizontal L1445
  constraint vertical L1446
  constraint horizontal L1448
  constraint vertical L1447
  constraint horizontal L1450
  constraint vertical L1449
sketch "Sketch2" plane through (0, 0, 0) normal (0, 0, 1) x (1, 0, 0)
sketch "botnplata" plane through (0, 0, 0) normal (0, 0, 1) x (1, 0, 0)
  line L0 (0, 0) -> (200, 0)
  line L1 (200, 0) -> (200, 100)
  line L2 (200, 100) -> (0, 100)
  line L3 (0, 100) -> (0, 0)
  dimension "d216" = 200
  dimension "d217" = 100
  constraint horizontal L0
  constraint vertical L1
  constraint horizontal L2
  constraint vertical L3
  constraint coincident L0.start L3.end
  measures "d216" distance of L0.start L0.end
  measures "d217" distance of L0.start L2.end
extrude "Extrude1" add sketch "botnplata" along normal blind 4 makes body 1
sketch "botnplata fremri fingur sketch" plane through (0, 0, 0) normal (0, -1, 0) x (1, 0, 0)
  line L0 (0, 0) -> (200, 0)
  line L1 (200, 0) -> (200, 4)
  line L2 (200, 4) -> (0, 4)
  line L3 (0, 4) -> (0, 0)
  line L4 (6.4516, 0) -> (12.9032, 0)
  line L5 (12.9032, 0) -> (12.9032, 4)
  line L6 (12.9032, 4) -> (6.4516, 4)
  line L7 (6.4516, 4) -> (6.4516, 0)
  dimension "d222" = 6.4516
  dimension "d223" = 6.4516
  constraint horizontal L4
  constraint vertical L5
  constraint horizontal L6
  constraint vertical L7
  constraint coincident L2 L5.end
  constraint coincident L0 L4.start
  measures "d222" distance of L5.end L6.end
  measures "d223" distance of L3 L7
extrude "Extrude2" cut sketch "botnplata fremri fingur sketch" against normal blind 4 contours L0 L2 L4 L5 L6 L7 bodies 1
pattern_linear "R-Pattern1" count 15 spacing 12.9032 along (1, 0, 0) of "Extrude2"
sketch "Sketch6" plane through (0, 0, 0) normal (0, 1, 0) x (1, 0, 0)
  line L0 (0, 0) -> (200, 0)
  line L1 (200, 0) -> (200, -96.5685)
  line L2 (200, -96.5685) -> (0, -96.5685)
  line L3 (0, -96.5685) -> (0, 0)
  dimension "d230" = 96.5685
  dimension "d430" = 200
  constraint perpendicular L0 L1
  constraint parallel L0 L2
  constraint parallel L1 L3
  constraint horizontal L0
  constraint coincident L0.start L3.end
  measures "d230" distance of L0.start L2.end
  measures "d430" distance of L1 L3
extrude "Extrude3" add sketch "Sketch6" along normal blind 4 separate body makes body 2
combine "Combine1" operation cut target body 2 tool bodies 1 keep tools
sketch "Sketch7" plane through (0, 0, 0) normal (-1, 0, 0) x (0, -1, 0)
  line L0 (-4, 4) -> (0, 4)
  line L1 (0, 4) -> (0, 96.5685)
  line L2 (0, 96.5685) -> (-4, 96.5685)
  line L3 (-4, 96.5685) -> (-4, 4)
  line L4 (-4, 7.4283) -> (0, 7.4283)
  line L5 (0, 7.4283) -> (0, 14.8567)
  line L6 (0, 14.8567) -> (-4, 14.8567)
  line L7 (-4, 14.8567) -> (-4, 7.4283)
  dimension "d233" = 7.4283
  dimension "d241" = 7.4283
  constraint horizontal L4
  constraint vertical L5
  constraint horizontal L6
  constraint vertical L7
  constraint coincident L1 L5.end
  constraint coincident L3 L4.start
  measures "d233" distance of L4.start L6.end
  measures "d241" distance of origin L4
extrude "Extrude4" cut sketch "Sketch7" against normal blind 4 contours L1 L3 L4 L5 L6 L7 bodies 2
pattern_linear "R-Pattern2" count 6 spacing 14.8567 along (0, 0, 1) of "Extrude4"
fillet "Fillet1" radius 40 1 edges at (200, 2, 96.5685) on bodies 2
sketch "Sketch8" plane through (200, 0, 0) normal (1, 0, 0) x (0, 1, 0)
  line L0 (4, 56.5685) -> (0, 56.5685)
  line L1 (0, 56.5685) -> (0, 4)
  line L2 (4, 4) -> (4, 56.5685)
  line L3 (4, 7.4283) -> (0, 7.4283)
  line L4 (0, 7.4283) -> (0, 14.8567)
  line L5 (0, 14.8567) -> (4, 14.8567)
  line L6 (4, 14.8567) -> (4, 7.4283)
  line L7 (0, 4) -> (4, 4)
  dimension "d245" = 7.4283
  dimension "d246" = 7.4283
  constraint horizontal L3
  constraint vertical L4
  constraint horizontal L5
  constraint vertical L6
  constraint coincident L1 L4.end
  constraint coincident L2 L3.start
  measures "d245" distance of L3.end L4.end
  measures "d246" distance of origin L3
extrude "Extrude5" cut sketch "Sketch8" against normal blind 4 contours L1 L2 L3 L4 L5 L6 bodies 2
pattern_linear "R-Pattern3" count 4 spacing 11.4278 along (0, 0, 1) of "Extrude5"
extrude "Extrude6" add 1 faces at (82.6237, 4, 60.7601) along direction (0, -1, 0) blind 4 from surface at -96 separate body on bodies 2 makes body 3
combine "Combine2" operation cut target body 1 tool bodies 3 keep tools
sketch "Sketch9" plane through (0, 0, 0) normal (-1, 0, 0) x (0, -1, 0)
  line L0 (-100, 0) -> (0, 0)
  line L1 (0, 0) -> (0, 4)
  line L2 (0, 4) -> (-100, 4)
  line L3 (-100, 4) -> (-100, 0)
  line L4 (-86.6667, 4) -> (-93.3333, 4)
  line L5 (-93.3333, 4) -> (-93.3333, 0)
  line L6 (-93.3333, 0) -> (-86.6667, 0)
  line L7 (-86.6667, 0) -> (-86.6667, 4)
  dimension "d256" = 6.6667
  dimension "d257" = 6.6667
  constraint horizontal L4
  constraint vertical L5
  constraint horizontal L6
  constraint vertical L7
  constraint coincident L0 L5.end
  constraint coincident L2 L4.start
  measures "d256" distance of L4.start L4.end
  measures "d257" distance of L3 L5
extrude "Extrude7" cut sketch "Sketch9" against normal blind 4 contours L0 L2 L4 L5 L6 L7 bodies 1
pattern_linear "R-Pattern4" count 7 spacing 13.3333 along (0, -1, 0) of "Extrude7"
sketch "bakplata sketch" plane through (0, 0, 0) normal (1, 0, 0) x (0, 1, 0)
  line L0 (0, 0) -> (100, 0)
  line L1 (100, 0) -> (100, 96.5685)
  line L2 (100, 96.5685) -> (0, 96.5685)
  line L3 (0, 96.5685) -> (0, 0)
  dimension "d264" = 100
  dimension "d265" = 96.5685
  constraint perpendicular L0 L1
  constraint parallel L0 L2
  constraint parallel L1 L3
  constraint horizontal L0
  constraint coincident L0.start L3.end
  measures "d264" distance of L0.start L0.end
  measures "d265" distance of L0.start L2.end
extrude "Extrude8" add sketch "bakplata sketch" along normal blind 4 separate body makes body 4
combine "Combine3" operation cut target body 4 tool bodies 2 1 3 keep tools
sketch "fremri plata fingur sketch" plane through (200, 0, 0) normal (1, 0, 0) x (0, 1, 0)
  line L0 (0, 0) -> (100, 0)
  line L1 (100, 0) -> (100, 4)
  line L2 (100, 4) -> (0, 4)
  line L3 (0, 4) -> (0, 0)
  line L4 (13.3333, 4) -> (6.6667, 4)
  line L5 (6.6667, 4) -> (6.6667, 0)
  line L6 (6.6667, 0) -> (13.3333, 0)
  line L7 (13.3333, 0) -> (13.3333, 4)
  dimension "d268" = 6.6667
  dimension "d269" = 6.6667
  constraint horizontal L4
  constraint vertical L5
  constraint horizontal L6
  constraint vertical L7
  constraint coincident L0 L5.end
  constraint coincident L2 L4.start
  measures "d268" distance of L4.start L4.end
  measures "d269" distance of L3 L5
extrude "Extrude9" cut sketch "fremri plata fingur sketch" against normal blind 4 contours L0 L2 L4 L5 L6 L7 bodies 1
pattern_linear "R-Pattern5" count 7 spacing 13.3333 along (0, 1, 0) of "Extrude9"
sketch "fremri plata" plane through (200, 0, 0) normal (1, 0, 0) x (0, 1, 0)
  line L0 (0, 41.7118) -> (0, 37.7124)
  line L1 (0, 0) -> (100, 0)
  line L2 (100, 0) -> (100, 56.5685)
  line L3 (100, 56.5685) -> (0, 56.5685)
  line L4 (0, 56.5685) -> (0, 0)
  line L5 (4, 37.7124) -> (4, 41.7118)
  line L6 (4, 41.7118) -> (0, 41.7118)
  line L7 (0, 37.7124) -> (4, 37.7124)
  dimension "d276" = 56.5685
  dimension "d561" = 100
  constraint perpendicular L1 L2
  constraint parallel L1 L3
  constraint parallel L2 L4
  constraint horizontal L1
  constraint coincident L1.start L4.end
  measures "d276" distance of L1.start L3.end
  measures "d561" distance of L2.end L3.end
extrude "Extrude10" add sketch "fremri plata" against normal blind 4 separate body makes body 5
combine "Combine4" operation cut target body 5 tool bodies 3 1 2 keep tools
sketch "milliplata" plane through (0, 0, 0) normal (0, 0, 1) x (1, 0, 0)
  line L0 (0, 0) -> (4, 0)
  line L1 (4, 0) -> (143.4315, 0)
  line L2 (143.4315, 0) -> (143.4315, 100)
  line L3 (143.4315, 100) -> (4, 100)
  line L4 (4, 100) -> (4, 0)
  dimension "d280" = 4
  dimension "d281" = 100
  dimension "d282" = 139.4315
  constraint coincident L0.start origin
  constraint horizontal L0
  constraint perpendicular L1 L2
  constraint parallel L1 L3
  constraint parallel L2 L4
  constraint parallel L0 L1
  measures "d280" distance of L0.start L0.end
  measures "d281" distance of L0.end L3.end
  measures "d282" distance of L0.end L1.end
extrude "Extrude11" add sketch "milliplata" along normal blind 4 from surface at 9 separate body makes body 6
sketch "milliplata fingur 1" plane through (0, 0, 0) normal (0, -1, 0) x (1, 0, 0)
  line L0 (4, 9) -> (143.4315, 9)
  line L1 (143.4315, 9) -> (143.4315, 13)
  line L2 (143.4315, 13) -> (4, 13)
  line L3 (4, 13) -> (4, 9)
  line L4 (4, 9) -> (13.1765, 9)
  line L5 (13.1765, 9) -> (13.1765, 13)
  line L6 (13.1765, 13) -> (4, 13)
  line L7 (4, 13) -> (4, 9)
  dimension "d288" = 9.1765
  constraint horizontal L4
  constraint vertical L5
  constraint horizontal L6
  constraint vertical L7
  constraint coincident L2 L5.end
  constraint coincident L0.start L3.end
  measures "d288" distance of L5.end L2.end
extrude "Extrude12" cut sketch "milliplata fingur 1" against normal blind 4 contours L0 L2 L3 L4 L5 L6 L7 bodies 6
pattern_linear "R-Pattern6" count 8 spacing 18.8571 along (1, 0, 0) of "Extrude12"
sketch "milliplata fingur 2" plane through (0, 100, 0) normal (0, 1, 0) x (-1, 0, 0)
  line L0 (-143.4315, 9) -> (-4, 9)
  line L1 (-4, 9) -> (-4, 13)
  line L2 (-4, 13) -> (-143.4315, 13)
  line L3 (-143.4315, 13) -> (-143.4315, 9)
  line L4 (-4, 9) -> (-13.1765, 9)
  line L5 (-13.1765, 9) -> (-13.1765, 13)
  line L6 (-13.1765, 13) -> (-4, 13)
  line L7 (-4, 13) -> (-4, 9)
  dimension "d295" = 9.1765
  constraint horizontal L4
  constraint vertical L5
  constraint horizontal L6
  constraint vertical L7
  constraint coincident L2 L5.end
  constraint coincident L0.end L1.start
  measures "d295" distance of L5.end L1.end
extrude "Extrude13" cut sketch "milliplata fingur 2" against normal blind 4 contours L0 L1 L2 L4 L5 L6 L7 bodies 6
pattern_linear "R-Pattern7" count 8 spacing 18.8571 along (1, 0, 0) of "Extrude13"
combine "Combine5" operation cut target body 2 tool bodies 6 keep tools
combine "Combine6" operation cut target body 3 tool bodies 6 keep tools
extrude "Extrude25" add 1 faces at (132.7731, 97.3333, 13) along direction (0, 0, -1) up to surface (4 mm away) on bodies 3 bodies 3
extrude "Extrude26" add 1 faces at (132.7731, 1.3333, 9) along direction (0, 0, 1) up to surface (4 mm away) on bodies 2 bodies 2
sketch "Sketch42" plane through (0, 0, 0) normal (0, 1, 0) x (1, 0, 0)
  line L0 (0, 0) -> (200, 0)
  line L1 (200, 0) -> (200, -48.5685)
  line L2 (200, -48.5685) -> (196, -48.5685)
  line L3 (200, 0) -> (151.4315, 0)
  line L4 (151.4315, 0) -> (151.4315, -4)
  dimension "d587" = 200
  dimension "d588" = 48.5685
  dimension "d589" = 4
  dimension "d590" = 48.5685
  dimension "d591" = 4
  constraint coincident L0.start origin
  constraint horizontal L0
  constraint perpendicular L0 L1
  constraint perpendicular L1 L2
  constraint coincident L0 L3.end
  constraint perpendicular L0 L4
  measures "d587" distance of L0.start L0.end
  measures "d588" distance of L0.end L1.end
  measures "d589" distance of L1.end L2.end
  measures "d590" distance of L0.end L3.end
  measures "d591" distance of L3.end L4.end
sketch "rail+guide" plane through (0, 0, 0) normal (0, 1, 0) x (1, 0, 0)
  line L0 (0, 0) -> (200, 0)
  line L1 (200, 0) -> (143.4315, -56.5685)
  line L2 (200, 0) -> (236, 0) construction
  circle A0 centre (143.4315, -56.5685) radius 43.5685
  line L3 (200, 0) -> (151.9167, -48.0833)
  circle A1 centre (151.9167, -48.0833) radius 44.5685
  line L4 (200, 0) -> (200, -4)
  line L5 (200, -4) -> (196, -4)
  line L6 (196, -4) -> (196, -100.5685)
  line L7 (196, -4) -> (99.4315, -4)
  line L8 (187, -56.5685) -> (143.4315, -56.5685)
  line L9 (143.4315, -56.5685) -> (184.8676, -43.1051)
  line L10 (143.4315, -56.5685) -> (187, -56.5685) construction
  line L11 (187, -56.5685) -> (184.8676, -43.1051)
  line L12 (184.8676, -43.1051) -> (188.8184, -42.4794)
  line L13 (188.8184, -42.4794) -> (190.9508, -55.9428)
  line L14 (190.9508, -55.9428) -> (187, -56.5685)
  line L15 (0, 0) -> (157.5736, 0)
  dimension "d431" = 200
  dimension "d432" = 135
  dimension "d433" = 80
  dimension "d434" = 87.1371
  dimension "d435" = 68
  dimension "d436" = 89.1371
  dimension "d437" = 4
  dimension "d438" = 4
  dimension "d460" = 43.5685
  dimension "d461" = 18
  dimension "d462" = 4
  dimension "d563" = 29.5
  dimension "d592" = 96.5685
  dimension "d593" = 96.5685
  constraint coincident L0.start L15.start
  constraint horizontal L0
  constraint horizontal L2
  constraint coincident L1.end A0.centre
  constraint parallel L1 L3
  constraint coincident L3.end A1.centre
  constraint perpendicular L0 L4
  constraint perpendicular L4 L5
  constraint perpendicular L5 L6
  constraint perpendicular L6 L7
  constraint coincident A0 L8.start
  constraint horizontal L8
  constraint horizontal L10
  constraint perpendicular L11 L12
  constraint parallel L11 L13
  constraint parallel L12 L14
  constraint parallel L0 L15
  measures "d431" distance of L0.start L0.end
  measures "d432" angle of L1 L2
  measures "d433" distance of L0.end L1.end
  measures "d434" diameter of A0
  measures "d435" distance of L0.end L3.end
  measures "d436" diameter of A1
  measures "d437" distance of L0.end L4.end
  measures "d438" distance of L4.end L5.end
  measures "d460" distance of L1.end L9.end
  measures "d461" angle of L9 L10
  measures "d462" distance of L8.start L13.end
  measures "d592" distance of L5.end L6.end
  measures "d593" distance of L5.end L7.end
extrude "Extrude43" add sketch "rail+guide" along normal blind 4 from surface at 4 separate body contours L1 L3 A1 L6 | L1 L3 A1 L7 makes body 7
extrude "Extrude44" add 1 faces at (186.1995, 8, 11.1282) along direction (0, -1, 0) blind 4 from surface at -88 separate body on bodies 7 makes body 8
sketch "hola" plane through (0, 0, 0) normal (0, 1, 0) x (1, 0, 0)
  line L0 (0, 0) -> (192, 0)
  line L1 (192, 0) -> (192, -8)
  line L2 (190, -6) -> (194, -6)
  line L3 (194, -6) -> (194, -10)
  line L4 (194, -10) -> (190, -10)
  line L5 (190, -10) -> (190, -6)
  line L6 (190, -6) -> (194, -10) construction
  line L7 (194, -6) -> (190, -10) construction
  point P0 (192, -8)
  dimension "d445" = 192
  dimension "d446" = 8
  dimension "d447" = 4
  dimension "d448" = 4
  constraint coincident L0.start origin
  constraint horizontal L0
  constraint perpendicular L0 L1
  constraint horizontal L2
  constraint perpendicular L2 L3
  constraint parallel L2 L4
  constraint parallel L3 L5
  constraint coincident L6 P0
  constraint coincident L7 P0
  constraint coincident P0 L1.end
  measures "d445" distance of L0.start L0.end
  measures "d446" distance of L0.end P0
  measures "d447" distance of L3.end L4.end
  measures "d448" distance of L2.end L3.end
extrude "Extrude45" cut sketch "hola" along normal through all bodies 2 7 8
extrude "Extrude48" add sketch "rail+guide" along normal blind 100 separate body contours A0 L12 L13 L14 | A0 L11 makes body 9
sketch "fingur_guide" plane through (0, 100, 0) normal (0, 1, 0) x (-1, 0, 0)
  line L0 (-190.9508, 55.9428) -> (-188.8184, 42.4794)
  line L1 (-188.8184, 42.4794) -> (-184.8676, 43.1051)
  line L2 (-184.8676, 43.1051) -> (-187, 56.5685)
  line L3 (-187, 56.5685) -> (-190.9508, 55.9428)
  line L4 (-187, 56.5685) -> (-190.9508, 55.9428)
  line L5 (-190.9508, 55.9428) -> (-190.24, 51.455)
  line L6 (-190.24, 51.455) -> (-186.2892, 52.0807)
  line L7 (-186.2892, 52.0807) -> (-187, 56.5685)
  dimension "d469" = 4.5437
  constraint perpendicular L4 L5
  constraint parallel L4 L6
  constraint parallel L5 L7
  constraint coincident L0.start L3.end
  constraint perpendicular L0 L4
  constraint coincident L2.end L3.start
  measures "d469" distance of L2.end L6.end
extrude "Extrude49" cut sketch "fingur_guide" against normal blind 4 contours L0 L2 L3 L4 L5 L6 L7 bodies 9
pattern_linear "R-Pattern15" count 2 spacing 9.1816 along (-0.156434, 0, -0.987688) of "Extrude49"
extrude "Extrude50" cut 2 faces at (189.16, 96, 53.1595) (186.6486, 96, 45.8264) along direction (0, 1, 0) blind 4 from surface at -96 on bodies 9 bodies 9
pattern_path "PathPattern2" count 5 spacing 13.6875 from (186.4636, 0, 49.7529) turning path "rail+guide" along A0 of bodies 9 makes body 10 at (181.4011, 65.3333, 36.3017) makes body 11 at (173.2799, 65.3333, 25.5604) makes body 12 at (163.6144, 65.3333, 18.5562) makes body 13 at (150.8801, 34.6667, 14.1798)